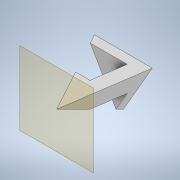
# Autodesk Inventor part: Деталь2Инди1
Saved by Autodesk Inventor 2021.1 (Build 251245010, 245A)
## iProperties
Created: 2023-10-25
Part Number: Деталь2Инди1
Material: Типовые
Document SubType Name: Modeling
Designer: Lenovo
Density: 1 g/cm^3
Appearance: По умолчанию
Author: Lenovo
Autodesk Inventor part; units mm, degrees
ref_plane "YZ Plane" through (0, 0, 0) normal (1, 0, 0) x (0, 1, 0)
ref_plane "XZ Plane" through (0, 0, 0) normal (0, 1, 0) x (-1, 0, 0)
sketch "Эскиз1" plane through (0, 0, 0) normal (0, 0, 1) x (1, 0, 0)
  circle A0 centre (0, 0) radius 45
  line L0 (0, -45) -> (-38.9711, 22.5)
  line L1 (-38.9711, 22.5) -> (38.9711, 22.5)
  line L2 (38.9711, 22.5) -> (0, -45)
  dimension "d0" = 90
  constraints: 6 end point, 2 coincident, 1 vertical alignment, 9 other
ref_plane "РабПлоскость1" through (0, 0, 90) normal (0, 0, 1) x (1, 0, 0)
sketch "Эскиз5" plane through (0, 0, 0) normal (0, 1, 0) x (-1, 0, 0)
  point P0 (0, 0)
sketch "Эскиз6" plane through (0, 0, 0) normal (1, 0, 0) x (0, 1, 0)
  point P0 (0, 0)
sketch "Эскиз7" plane through (0, 0, 0) normal (0, 1, 0) x (-1, 0, 0)
  point P0 (0, 0)
sketch "Эскиз8" plane through (0, 0, 90) normal (0, 0, 1) x (1, 0, 0)
  point P0 (0, 0)
loft "Лофт2" add profiles "Эскиз1" section 1 point at (0, 0, 90) contours L2 L0 L1
sketch "Эскиз9" plane through (0, 0, 0) normal (0, 1, 0) x (-1, 0, 0)
  point P0 (0, 0)
sketch "Эскиз10" plane through (0, 0, 0) normal (0, 1, 0) x (-1, 0, 0)
  line L0 (0, 10) -> (34.641, 10)
  line L1 (0, 90) -> (38.9711, 0) projected
  line L2 (0, 45) -> (19.4856, 45)
  line L3 (0, 45) -> (-15.1554, 10)
  line L4 (0, 90) -> (-38.9711, 0) projected
  line L5 (-15.1554, 10) -> (0, 10)
  line L6 (19.4856, 45) -> (34.641, 10)
  point P0 (0, 0)
  constraints: 10 end point, 1 collinear, 1 midpoint, 1 parallel, 1 point on line
extrude "Выдавливание1" cut sketch "Эскиз10" along normal mid plane 10000
